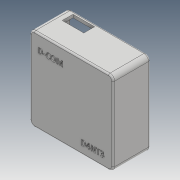
# Autodesk Inventor part: base
Saved by Autodesk Inventor 2017 (Build 210142000, 142)
## iProperties
Created: 2020-06-11
Part Number: base
Material: Generic
Document SubType Name: Modeling
Designer: c
Density: 1 g/cm^3
Appearance: Default
Author: c
Autodesk Inventor part; units mm, degrees
ref_plane "YZ Plane" through (0, 0, 0) normal (1, 0, 0) x (0, 1, 0)
ref_plane "XZ Plane" through (0, 0, 0) normal (0, 1, 0) x (-1, 0, 0)
ref_plane "XY Plane" through (0, 0, 0) normal (0, 0, 1) x (1, 0, 0)
sketch "Sketch1" plane through (0, 0, 0) normal (0, 1, 0) x (-1, 0, 0)
  line L0 (13, 15) -> (-37, 15)
  line L1 (-37, 15) -> (-37, -35)
  line L2 (-37, -35) -> (13, -35)
  line L3 (13, -35) -> (13, 15)
  line L4 (12, 17) -> (-36, 17)
  line L5 (-39, 14) -> (-39, -34)
  line L6 (-36, -37) -> (12, -37)
  line L7 (15, -34) -> (15, 14)
  arc A0 (15, 14) -> (12, 17) centre (12, 14) ccw
  arc A1 (-36, 17) -> (-39, 14) centre (-36, 14) ccw
  arc A2 (-39, -34) -> (-36, -37) centre (-36, -34) ccw
  arc A3 (12, -37) -> (15, -34) centre (12, -34) ccw
  point P0 (0, 0)
  dimension "d0" = 50
  dimension "d1" = 50
  dimension "d2" = 3
  constraints: 16 end point, 8 point on circle, 8 tangent, 4 centre point, 4 parallel, 3 equal radius, 2 perpendicular, 1 horizontal, 3 other
  measures "d0" distance of L2.end L1.end
  measures "d1" distance of L1.end L0.end
  measures "d2" radius of A0
extrude "Extrusion1" add sketch "Sketch1" along normal blind 24
sketch "Sketch2" plane through (0, 0, 0) normal (0, -1, 0) x (1, 0, 0)
  line L0 (36, 17) -> (-12, 17)
  line L1 (-15, 14) -> (-15, -34)
  line L2 (-12, -37) -> (36, -37)
  line L3 (39, -34) -> (39, 14)
  arc A0 (39, 14) -> (36, 17) centre (36, 14) ccw
  arc A1 (-12, 17) -> (-15, 14) centre (-12, 14) ccw
  arc A2 (-15, -34) -> (-12, -37) centre (-12, -34) ccw
  arc A3 (36, -37) -> (39, -34) centre (36, -34) ccw
  point P0 (0, 0)
  dimension "d5" = 3
  constraints: 8 end point, 8 point on circle, 8 tangent, 4 centre point, 3 equal radius, 2 parallel, 1 horizontal, 1 perpendicular
  measures "d5" radius of A0
extrude "Extrusion2" add sketch "Sketch2" against normal blind 2
fillet "Fillet1" radius 1 8 edges at (-14.1213, 0, 16.1213) (-15, 0, -10) (-14.1213, 0, -36.1213) (12, 0, -37) (38.1213, 0, -36.1213) (39, 0, -10) (38.1213, 0, 16.1213) (12, 0, 17)
sketch "Sketch3" plane through (36, 24, -37) normal (0, 0, -1) x (-1, 0, 0)
  line L0 (29, -12) -> (19, -12)
  line L1 (19, -12) -> (19, -8)
  line L2 (19, -8) -> (29, -8)
  line L3 (29, -8) -> (29, -12)
  line L4 (29, -18) -> (19, -18)
  line L5 (19, -18) -> (19, -14)
  line L6 (19, -14) -> (29, -14)
  line L7 (29, -14) -> (29, -18)
  line L8 (0, 0) -> (48, 0) projected
  line L9 (51, -23) -> (51, 0) projected
  line L10 (0, -24) -> (48, -24) projected
  point P0 (36, -24)
  dimension "d9" = 10
  dimension "d10" = 4
  dimension "d11" = 10
  dimension "d12" = 2
  dimension "d16" = 22
  dimension "d17" = 4
  dimension "d25" = 10
  constraints: 16 end point, 4 parallel, 2 horizontal, 2 perpendicular, 1 point on line
  measures "d9" distance of L1.end L2.end
  measures "d10" distance of L0.end L1.end
  measures "d11" distance of L5.end L6.end
  measures "d12" distance between parallel lines of L0 L6
  measures "d16" distance between parallel lines of L9 L7
  measures "d17" distance of L4.end L5.end
  measures "d25" distance between parallel lines of L10 L6
extrude "Extrusion3" cut sketch "Sketch3" against normal blind 4
sketch "Sketch4" plane through (0, 0, 0) normal (0, -1, 0) x (1, 0, 0)
  line L0 (18.0093, -28.2459) -> (38.9151, -28.2459) construction
  line L1 (38.9151, -28.2459) -> (38.9151, -38.6095) construction
  line L2 (38.9151, -38.6095) -> (18.0093, -38.6095) construction
  line L3 (18.0093, -38.6095) -> (18.0093, -28.2459) construction
  line L4 (-9.7906, 9.4463) -> (11.1152, 9.4463) construction
  line L5 (11.1152, 9.4463) -> (11.1152, -33.5941) construction
  line L6 (11.1152, -33.5941) -> (-9.7906, -33.5941) construction
  line L7 (-9.7906, -33.5941) -> (-9.7906, 9.4463) construction
  spline S0 degree 2 poles (21.2858, -29.9976) (21.2858, -30.4774) (21.0361, -31.1577) (20.5661, -31.5915) (19.8957, -31.7919) (19.4323, -31.7919) knots 0 0 0 1 2 3 4 4 4
  line L8 (19.4323, -31.7919) -> (18.6009, -31.7919)
  spline S1 degree 2 poles (18.6009, -31.7919) (18.5121, -31.7919) (18.3905, -31.6868) (18.3905, -31.5685) knots 0 0 0 1 2 2 2
  line L9 (18.3905, -31.5685) -> (18.3905, -28.5319)
  spline S2 degree 2 poles (18.3905, -28.5319) (18.3905, -28.4135) (18.5121, -28.3084) (18.6009, -28.3084) knots 0 0 0 1 2 2 2
  line L10 (18.6009, -28.3084) -> (19.4948, -28.3084)
  spline S3 degree 2 poles (19.4948, -28.3084) (19.9614, -28.3084) (20.6088, -28.5253) (21.0558, -28.9558) (21.2858, -29.5835) (21.2858, -29.9976) knots 0 0 0 1 2 3 4 4 4
  spline S4 degree 2 poles (20.553, -30.0239) (20.553, -29.7774) (20.4379, -29.3502) (20.1816, -29.038) (19.7807, -28.8638) (19.4553, -28.8638) knots 0 0 0 1 2 3 4 4 4
  line L11 (19.4553, -28.8638) -> (19.0971, -28.8638)
  line L12 (19.0971, -28.8638) -> (19.0971, -31.2333)
  line L13 (19.0971, -31.2333) -> (19.4652, -31.2333)
  spline S5 degree 2 poles (19.4652, -31.2333) (19.7577, -31.2333) (20.1553, -31.0821) (20.4215, -30.7797) (20.553, -30.3262) (20.553, -30.0239) knots 0 0 0 1 2 3 4 4 4
  spline S6 degree 2 poles (24.1713, -30.7929) (24.1713, -30.9309) (24.1154, -31.0722) (24.0661, -31.0722) knots 0 0 0 1 2 2 2
  line L14 (24.0661, -31.0722) -> (23.7572, -31.0722)
  line L15 (23.7572, -31.0722) -> (23.7572, -31.6999)
  spline S7 degree 2 poles (23.7572, -31.6999) (23.7572, -31.7262) (23.7243, -31.7689) (23.6455, -31.7952) (23.514, -31.8084) (23.4121, -31.8084) knots 0 0 0 1 2 3 4 4 4
  spline S8 degree 2 poles (23.4121, -31.8084) (23.3168, -31.8084) (23.1854, -31.7952) (23.1065, -31.7689) (23.0769, -31.7262) (23.0769, -31.6999) knots 0 0 0 1 2 3 4 4 4
  line L16 (23.0769, -31.6999) -> (23.0769, -31.0722)
  line L17 (23.0769, -31.0722) -> (21.7426, -31.0722)
  spline S9 degree 2 poles (21.7426, -31.0722) (21.7032, -31.0722) (21.6441, -31.0525) (21.6046, -30.9868) (21.5849, -30.8586) (21.5849, -30.7535) knots 0 0 0 1 2 3 4 4 4
  spline S10 degree 2 poles (21.5849, -30.7535) (21.5849, -30.668) (21.5915, -30.5431) (21.6112, -30.438) (21.6473, -30.3492) (21.6736, -30.2966) knots 0 0 0 1 2 3 4 4 4
  line L18 (21.6736, -30.2966) -> (22.7581, -28.3873)
  spline S11 degree 2 poles (22.7581, -28.3873) (22.7713, -28.361) (22.837, -28.3281) (22.952, -28.3018) (23.1295, -28.2919) (23.2577, -28.2919) knots 0 0 0 1 2 3 4 4 4
  spline S12 degree 2 poles (23.2577, -28.2919) (23.3957, -28.2919) (23.5863, -28.3051) (23.7046, -28.3347) (23.7572, -28.3774) (23.7572, -28.407) knots 0 0 0 1 2 3 4 4 4
  line L19 (23.7572, -28.407) -> (23.7572, -30.507)
  line L20 (23.7572, -30.507) -> (24.0661, -30.507)
  spline S13 degree 2 poles (24.0661, -30.507) (24.1088, -30.507) (24.1713, -30.6384) (24.1713, -30.7929) knots 0 0 0 1 2 2 2
  line L21 (23.0769, -28.9032) -> (23.0703, -28.9032)
  line L22 (23.0703, -28.9032) -> (22.1502, -30.507)
  line L23 (22.1502, -30.507) -> (23.0769, -30.507)
  line L24 (23.0769, -30.507) -> (23.0769, -28.9032)
  spline S14 degree 2 poles (27.5333, -31.5455) (27.5333, -31.6079) (27.4905, -31.7032) (27.4182, -31.7689) (27.3164, -31.7985) (27.2671, -31.7985) knots 0 0 0 1 2 3 4 4 4
  line L25 (27.2671, -31.7985) -> (26.9647, -31.7985)
  spline S15 degree 2 poles (26.9647, -31.7985) (26.8727, -31.7985) (26.7347, -31.7591) (26.6196, -31.6605) (26.5112, -31.4896) (26.4422, -31.3581) knots 0 0 0 1 2 3 4 4 4
  line L26 (26.4422, -31.3581) -> (25.5746, -29.7281)
  spline S16 degree 2 poles (25.5746, -29.7281) (25.499, -29.5835) (25.3445, -29.245) (25.2821, -29.0873) knots 0 0 0 1 2 2 2
  line L27 (25.2821, -29.0873) -> (25.2755, -29.0873)
  spline S17 degree 2 poles (25.2755, -29.0873) (25.2887, -29.2812) (25.2985, -29.6657) (25.2985, -29.8694) knots 0 0 0 1 2 2 2
  line L28 (25.2985, -29.8694) -> (25.2985, -31.6934)
  spline S18 degree 2 poles (25.2985, -31.6934) (25.2985, -31.7196) (25.2689, -31.7624) (25.1966, -31.7919) (25.0718, -31.8084) (24.9764, -31.8084) knots 0 0 0 1 2 3 4 4 4
  spline S19 degree 2 poles (24.9764, -31.8084) (24.8811, -31.8084) (24.7563, -31.7919) (24.6872, -31.7624) (24.661, -31.7196) (24.661, -31.6934) knots 0 0 0 1 2 3 4 4 4
  line L29 (24.661, -31.6934) -> (24.661, -28.5614)
  spline S20 degree 2 poles (24.661, -28.5614) (24.661, -28.4333) (24.8088, -28.3084) (24.9173, -28.3084) knots 0 0 0 1 2 2 2
  line L30 (24.9173, -28.3084) -> (25.2952, -28.3084)
  spline S21 degree 2 poles (25.2952, -28.3084) (25.3971, -28.3084) (25.5384, -28.3445) (25.6469, -28.4234) (25.7455, -28.568) (25.798, -28.6732) knots 0 0 0 1 2 3 4 4 4
  line L31 (25.798, -28.6732) -> (26.475, -29.945)
  spline S22 degree 2 poles (26.475, -29.945) (26.5342, -30.0633) (26.6492, -30.2868) (26.7577, -30.5103) (26.8595, -30.7239) (26.9088, -30.8323) knots 0 0 0 1 2 3 4 4 4
  line L32 (26.9088, -30.8323) -> (26.9121, -30.8323)
  spline S23 degree 2 poles (26.9121, -30.8323) (26.9023, -30.645) (26.8957, -30.2342) (26.8957, -30.0469) knots 0 0 0 1 2 2 2
  line L33 (26.8957, -30.0469) -> (26.8957, -28.4103)
  spline S24 degree 2 poles (26.8957, -28.4103) (26.8957, -28.384) (26.9286, -28.3412) (27.0041, -28.3084) (27.1257, -28.2952) (27.2243, -28.2952) knots 0 0 0 1 2 3 4 4 4
  spline S25 degree 2 poles (27.2243, -28.2952) (27.3164, -28.2952) (27.4379, -28.3084) (27.507, -28.3412) (27.5333, -28.384) (27.5333, -28.4103) knots 0 0 0 1 2 3 4 4 4
  line L34 (27.5333, -28.4103) -> (27.5333, -31.5455)
  spline S26 degree 2 poles (30.606, -28.5976) (30.606, -28.6765) (30.5929, -28.7882) (30.5666, -28.8539) (30.5239, -28.8868) (30.5009, -28.8868) knots 0 0 0 1 2 3 4 4 4
  line L35 (30.5009, -28.8868) -> (29.63, -28.8868)
  line L36 (29.63, -28.8868) -> (29.63, -31.6966)
  spline S27 degree 2 poles (29.63, -31.6966) (29.63, -31.7229) (29.5938, -31.7657) (29.5149, -31.7919) (29.3769, -31.8084) (29.275, -31.8084) knots 0 0 0 1 2 3 4 4 4
  spline S28 degree 2 poles (29.275, -31.8084) (29.1732, -31.8084) (29.0351, -31.7919) (28.9563, -31.7657) (28.9201, -31.7229) (28.9201, -31.6966) knots 0 0 0 1 2 3 4 4 4
  line L37 (28.9201, -31.6966) -> (28.9201, -28.8868)
  line L38 (28.9201, -28.8868) -> (28.0492, -28.8868)
  spline S29 degree 2 poles (28.0492, -28.8868) (28.0229, -28.8868) (27.9835, -28.8539) (27.9572, -28.7882) (27.9441, -28.6765) (27.9441, -28.5976) knots 0 0 0 1 2 3 4 4 4
  spline S30 degree 2 poles (27.9441, -28.5976) (27.9441, -28.5187) (27.9572, -28.4037) (27.9835, -28.338) (28.0229, -28.3084) (28.0492, -28.3084) knots 0 0 0 1 2 3 4 4 4
  line L39 (28.0492, -28.3084) -> (30.5009, -28.3084)
  spline S31 degree 2 poles (30.5009, -28.3084) (30.5239, -28.3084) (30.5666, -28.338) (30.5929, -28.4037) (30.606, -28.5187) (30.606, -28.5976) knots 0 0 0 1 2 3 4 4 4
  spline S32 degree 2 poles (33.2023, -30.7732) (33.2023, -31.0328) (33.0018, -31.437) (32.6469, -31.7131) (32.1506, -31.8544) (31.8581, -31.8544) knots 0 0 0 1 2 3 4 4 4
  spline S33 degree 2 poles (31.8581, -31.8544) (31.6807, -31.8544) (31.3685, -31.8018) (31.1286, -31.7295) (30.9708, -31.6473) (30.9248, -31.6046) (30.8985, -31.5488) (30.8788, -31.4765) (30.8722, -31.368) (30.8722, -31.2891) knots 0 0 0 1 2 3 4 5 6 7 8 8 8
  spline S34 degree 2 poles (30.8722, -31.2891) (30.8722, -31.1577) (30.9149, -31.0591) (30.9577, -31.0591) knots 0 0 0 1 2 2 2
  spline S35 degree 2 poles (30.9577, -31.0591) (30.984, -31.0591) (31.1187, -31.1314) (31.3225, -31.2168) (31.5985, -31.2891) (31.7727, -31.2891) knots 0 0 0 1 2 3 4 4 4
  spline S36 degree 2 poles (31.7727, -31.2891) (31.9206, -31.2891) (32.1473, -31.2201) (32.3051, -31.0919) (32.384, -30.9112) (32.384, -30.8027) knots 0 0 0 1 2 3 4 4 4
  spline S37 degree 2 poles (32.384, -30.8027) (32.384, -30.6812) (32.2887, -30.4873) (32.1046, -30.3492) (31.822, -30.2736) (31.6281, -30.2736) knots 0 0 0 1 2 3 4 4 4
  line L40 (31.6281, -30.2736) -> (31.3257, -30.2736)
  spline S38 degree 2 poles (31.3257, -30.2736) (31.2929, -30.2736) (31.2436, -30.2539) (31.2107, -30.1948) (31.1976, -30.0896) (31.1976, -30.0074) knots 0 0 0 1 2 3 4 4 4
  spline S39 degree 2 poles (31.1976, -30.0074) (31.1976, -29.9286) (31.2107, -29.83) (31.2403, -29.7774) (31.2863, -29.7544) (31.3192, -29.7544) knots 0 0 0 1 2 3 4 4 4
  line L41 (31.3192, -29.7544) -> (31.6248, -29.7544)
  spline S40 degree 2 poles (31.6248, -29.7544) (31.7825, -29.7544) (32.0257, -29.6821) (32.1901, -29.5473) (32.2755, -29.3567) (32.2755, -29.2384) knots 0 0 0 1 2 3 4 4 4
  spline S41 degree 2 poles (32.2755, -29.2384) (32.2755, -29.1497) (32.2164, -28.9919) (32.1013, -28.8769) (31.9173, -28.8079) (31.7924, -28.8079) knots 0 0 0 1 2 3 4 4 4
  spline S42 degree 2 poles (31.7924, -28.8079) (31.6511, -28.8079) (31.4046, -28.8901) (31.2074, -28.9919) (31.0694, -29.0774) (31.0365, -29.0774) knots 0 0 0 1 2 3 4 4 4
  spline S43 degree 2 poles (31.0365, -29.0774) (31.0168, -29.0774) (30.984, -29.0577) (30.961, -29.0051) (30.9511, -28.9032) (30.9511, -28.8211) knots 0 0 0 1 2 3 4 4 4
  spline S44 degree 2 poles (30.9511, -28.8211) (30.9511, -28.7553) (30.9577, -28.6666) (30.9741, -28.6074) (30.9971, -28.5647) (31.0497, -28.5121) (31.2173, -28.4103) (31.4703, -28.3117) (31.8023, -28.2459) (31.9962, -28.2459) knots 0 0 0 1 2 3 4 5 6 7 8 8 8
  spline S45 degree 2 poles (31.9962, -28.2459) (32.2492, -28.2459) (32.6403, -28.3642) (32.9065, -28.5877) (33.0445, -28.9131) (33.0445, -29.1201) knots 0 0 0 1 2 3 4 4 4
  spline S46 degree 2 poles (33.0445, -29.1201) (33.0445, -29.2779) (32.9624, -29.5506) (32.8079, -29.7675) (32.5713, -29.9187) (32.4201, -29.9549) knots 0 0 0 1 2 3 4 4 4
  line L42 (32.4201, -29.9549) -> (32.4201, -29.9647)
  spline S47 degree 2 poles (32.4201, -29.9647) (32.6009, -29.9844) (32.8933, -30.129) (33.0938, -30.3427) (33.2023, -30.6154) (33.2023, -30.7732) knots 0 0 0 1 2 3 4 4 4
  spline S48 degree 2 poles (-6.5141, 7.6946) (-6.5141, 7.2148) (-6.7638, 6.5345) (-7.2338, 6.1007) (-7.9042, 5.9002) (-8.3676, 5.9002) knots 0 0 0 1 2 3 4 4 4
  line L43 (-8.3676, 5.9002) -> (-9.1991, 5.9002)
  spline S49 degree 2 poles (-9.1991, 5.9002) (-9.2878, 5.9002) (-9.4094, 6.0054) (-9.4094, 6.1237) knots 0 0 0 1 2 2 2
  line L44 (-9.4094, 6.1237) -> (-9.4094, 9.1603)
  spline S50 degree 2 poles (-9.4094, 9.1603) (-9.4094, 9.2786) (-9.2878, 9.3838) (-9.1991, 9.3838) knots 0 0 0 1 2 2 2
  line L45 (-9.1991, 9.3838) -> (-8.3052, 9.3838)
  spline S51 degree 2 poles (-8.3052, 9.3838) (-7.8385, 9.3838) (-7.1911, 9.1669) (-6.7441, 8.7364) (-6.5141, 8.1087) (-6.5141, 7.6946) knots 0 0 0 1 2 3 4 4 4
  spline S52 degree 2 poles (-7.2469, 7.6683) (-7.2469, 7.9148) (-7.362, 8.342) (-7.6183, 8.6542) (-8.0192, 8.8284) (-8.3446, 8.8284) knots 0 0 0 1 2 3 4 4 4
  line L46 (-8.3446, 8.8284) -> (-8.7028, 8.8284)
  line L47 (-8.7028, 8.8284) -> (-8.7028, 6.4589)
  line L48 (-8.7028, 6.4589) -> (-8.3347, 6.4589)
  spline S53 degree 2 poles (-8.3347, 6.4589) (-8.0422, 6.4589) (-7.6446, 6.6101) (-7.3784, 6.9125) (-7.2469, 7.366) (-7.2469, 7.6683) knots 0 0 0 1 2 3 4 4 4
  spline S54 degree 2 poles (-4.7854, 7.2542) (-4.7854, 7.0998) (-4.8446, 6.9749) (-4.9103, 6.9749) knots 0 0 0 1 2 2 2
  line L49 (-4.9103, 6.9749) -> (-6.0277, 6.9749)
  spline S55 degree 2 poles (-6.0277, 6.9749) (-6.0967, 6.9749) (-6.1559, 7.1031) (-6.1559, 7.2542) knots 0 0 0 1 2 2 2
  spline S56 degree 2 poles (-6.1559, 7.2542) (-6.1559, 7.4054) (-6.0967, 7.5303) (-6.0277, 7.5303) knots 0 0 0 1 2 2 2
  line L50 (-6.0277, 7.5303) -> (-4.9103, 7.5303)
  spline S57 degree 2 poles (-4.9103, 7.5303) (-4.8775, 7.5303) (-4.8314, 7.504) (-4.7986, 7.4383) (-4.7854, 7.3298) (-4.7854, 7.2542) knots 0 0 0 1 2 3 4 4 4
  spline S58 degree 2 poles (-1.8343, 6.4294) (-1.8343, 6.3636) (-1.8408, 6.2683) (-1.8573, 6.2026) (-1.8868, 6.1533) (-1.946, 6.0909) (-2.1136, 5.9923) (-2.3601, 5.9035) (-2.6756, 5.8444) (-2.8563, 5.8444) knots 0 0 0 1 2 3 4 5 6 7 8 8 8
  spline S59 degree 2 poles (-2.8563, 5.8444) (-3.2145, 5.8444) (-3.7929, 6.0646) (-4.1939, 6.5049) (-4.4108, 7.1589) (-4.4108, 7.596) knots 0 0 0 1 2 3 4 4 4
  spline S60 degree 2 poles (-4.4108, 7.596) (-4.4108, 8.0397) (-4.1742, 8.7298) (-3.7469, 9.1965) (-3.1521, 9.4397) (-2.7939, 9.4397) knots 0 0 0 1 2 3 4 4 4
  spline S61 degree 2 poles (-2.7939, 9.4397) (-2.6493, 9.4397) (-2.3798, 9.3904) (-2.1498, 9.3115) (-1.969, 9.2096) (-1.8967, 9.1373) (-1.8671, 9.088) (-1.8507, 9.0125) (-1.8441, 8.9106) (-1.8441, 8.835) knots 0 0 0 1 2 3 4 5 6 7 8 8 8
  spline S62 degree 2 poles (-1.8441, 8.835) (-1.8441, 8.7561) (-1.854, 8.6411) (-1.8803, 8.5721) (-1.9197, 8.5392) (-1.9427, 8.5392) knots 0 0 0 1 2 3 4 4 4
  spline S63 degree 2 poles (-1.9427, 8.5392) (-1.9854, 8.5392) (-2.107, 8.6345) (-2.3042, 8.7495) (-2.577, 8.8448) (-2.7643, 8.8448) knots 0 0 0 1 2 3 4 4 4
  spline S64 degree 2 poles (-2.7643, 8.8448) (-2.9714, 8.8448) (-3.2967, 8.674) (-3.5268, 8.3617) (-3.6451, 7.9148) (-3.6451, 7.6355) knots 0 0 0 1 2 3 4 4 4
  spline S65 degree 2 poles (-3.6451, 7.6355) (-3.6451, 7.3265) (-3.5202, 6.8796) (-3.2836, 6.5871) (-2.9549, 6.4458) (-2.7479, 6.4458) knots 0 0 0 1 2 3 4 4 4
  spline S66 degree 2 poles (-2.7479, 6.4458) (-2.5573, 6.4458) (-2.2845, 6.5345) (-2.0873, 6.643) (-1.9591, 6.7284) (-1.9263, 6.7284) knots 0 0 0 1 2 3 4 4 4
  spline S67 degree 2 poles (-1.9263, 6.7284) (-1.9, 6.7284) (-1.8671, 6.7054) (-1.8441, 6.643) (-1.8343, 6.5279) (-1.8343, 6.4294) knots 0 0 0 1 2 3 4 4 4
  spline S68 degree 2 poles (1.8103, 7.6815) (1.8103, 7.2477) (1.5934, 6.5641) (1.1695, 6.0876) (0.5418, 5.8378) (0.131, 5.8378) knots 0 0 0 1 2 3 4 4 4
  spline S69 degree 2 poles (0.131, 5.8378) (-0.2765, 5.8378) (-0.8845, 6.0514) (-1.2887, 6.4852) (-1.4892, 7.1589) (-1.4892, 7.619) knots 0 0 0 1 2 3 4 4 4
  spline S70 degree 2 poles (-1.4892, 7.619) (-1.4892, 8.043) (-1.2723, 8.72) (-0.8483, 9.1932) (-0.2206, 9.4463) (0.1934, 9.4463) knots 0 0 0 1 2 3 4 4 4
  spline S71 degree 2 poles (0.1934, 9.4463) (0.5911, 9.4463) (1.1958, 9.2359) (1.6033, 8.7988) (1.8103, 8.135) (1.8103, 7.6815) knots 0 0 0 1 2 3 4 4 4
  spline S72 degree 2 poles (1.0676, 7.6453) (1.0676, 7.9181) (0.9822, 8.3683) (0.7751, 8.6904) (0.4301, 8.8646) (0.1704, 8.8646) knots 0 0 0 1 2 3 4 4 4
  spline S73 degree 2 poles (0.1704, 8.8646) (-0.0925, 8.8646) (-0.4408, 8.6674) (-0.6577, 8.3387) (-0.7465, 7.9017) (-0.7465, 7.6552) knots 0 0 0 1 2 3 4 4 4
  spline S74 degree 2 poles (-0.7465, 7.6552) (-0.7465, 7.3693) (-0.661, 6.9157) (-0.454, 6.5937) (-0.1089, 6.4228) (0.1507, 6.4228) knots 0 0 0 1 2 3 4 4 4
  spline S75 degree 2 poles (0.1507, 6.4228) (0.4136, 6.4228) (0.762, 6.6167) (0.9789, 6.9519) (1.0676, 7.3955) (1.0676, 7.6453) knots 0 0 0 1 2 3 4 4 4
  spline S76 degree 2 poles (6.4671, 5.9955) (6.4671, 5.9693) (6.4376, 5.9265) (6.3587, 5.9002) (6.2305, 5.8838) (6.1319, 5.8838) knots 0 0 0 1 2 3 4 4 4
  spline S77 degree 2 poles (6.1319, 5.8838) (6.0333, 5.8838) (5.9052, 5.9002) (5.8296, 5.9265) (5.7967, 5.9693) (5.7967, 5.9955) knots 0 0 0 1 2 3 4 4 4
  line L51 (5.7967, 5.9955) -> (5.7967, 8.8317)
  line L52 (5.7967, 8.8317) -> (5.7902, 8.8317)
  line L53 (5.7902, 8.8317) -> (4.7812, 5.9988)
  spline S78 degree 2 poles (4.7812, 5.9988) (4.7714, 5.966) (4.7221, 5.92) (4.6399, 5.8904) (4.5085, 5.8838) (4.4164, 5.8838) knots 0 0 0 1 2 3 4 4 4
  spline S79 degree 2 poles (4.4164, 5.8838) (4.3277, 5.8838) (4.1963, 5.897) (4.1141, 5.9265) (4.0648, 5.9693) (4.0582, 5.9988) knots 0 0 0 1 2 3 4 4 4
  line L54 (4.0582, 5.9988) -> (3.0822, 8.8317)
  line L55 (3.0822, 8.8317) -> (3.0756, 8.8317)
  line L56 (3.0756, 8.8317) -> (3.0756, 5.9955)
  spline S80 degree 2 poles (3.0756, 5.9955) (3.0756, 5.9693) (3.046, 5.9265) (2.9639, 5.9002) (2.839, 5.8838) (2.7404, 5.8838) knots 0 0 0 1 2 3 4 4 4
  spline S81 degree 2 poles (2.7404, 5.8838) (2.6418, 5.8838) (2.5136, 5.9002) (2.4348, 5.9265) (2.4052, 5.9693) (2.4052, 5.9955) knots 0 0 0 1 2 3 4 4 4
  line L57 (2.4052, 5.9955) -> (2.4052, 9.1012)
  spline S82 degree 2 poles (2.4052, 9.1012) (2.4052, 9.2392) (2.5498, 9.3838) (2.6714, 9.3838) knots 0 0 0 1 2 2 2
  line L58 (2.6714, 9.3838) -> (3.1348, 9.3838)
  spline S83 degree 2 poles (3.1348, 9.3838) (3.2596, 9.3838) (3.4371, 9.3444) (3.5653, 9.2491) (3.6507, 9.0946) (3.6836, 8.9829) knots 0 0 0 1 2 3 4 4 4
  line L59 (3.6836, 8.9829) -> (4.4394, 6.9059)
  line L60 (4.4394, 6.9059) -> (4.4493, 6.9059)
  line L61 (4.4493, 6.9059) -> (5.2315, 8.9763)
  spline S84 degree 2 poles (5.2315, 8.9763) (5.2676, 9.0913) (5.3498, 9.2458) (5.4615, 9.3444) (5.6094, 9.3838) (5.7113, 9.3838) knots 0 0 0 1 2 3 4 4 4
  line L62 (5.7113, 9.3838) -> (6.1878, 9.3838)
  spline S85 degree 2 poles (6.1878, 9.3838) (6.2601, 9.3838) (6.3653, 9.3477) (6.431, 9.2721) (6.4671, 9.1669) (6.4671, 9.1012) knots 0 0 0 1 2 3 4 4 4
  line L63 (6.4671, 9.1012) -> (6.4671, 5.9955)
  point P0 (0, 0)
  constraints: 4 other
emboss "Emboss1" sketch "Sketch4" operation cut depth 1 direction (0, 1, 0)
sketch "Sketch5" plane through (-12, 24, 17) normal (0, 0, 1) x (1, 0, 0)
  line L0 (29, -12) -> (29, -8) projected
  line L1 (17, -9) -> (2.9977, -9)
  line L2 (2.9977, -9) -> (2.9977, -2)
  line L3 (2.9977, -2) -> (17, -2)
  line L4 (17, -2) -> (17, -9)
  line L5 (-3, -23) -> (-3, 0) projected
  line L6 (0, -24) -> (48, -24) projected
  point P0 (12, -24)
  dimension "d26" = 20
  dimension "d27" = 15
  dimension "d28" = 7
  constraints: 8 end point, 2 parallel, 1 horizontal, 1 perpendicular
  measures "d26" distance between parallel lines of L5 L4
  measures "d27" distance between parallel lines of L6 L1
  measures "d28" distance between parallel lines of L1 L3
extrude "Extrusion4" cut sketch "Sketch5" against normal blind 4
fillet "Fillet2" radius 1 8 edges at (38.1213, 24, 16.1213) (39, 24, -10) (38.1213, 24, -36.1213) (12, 24, -37) (-14.1213, 24, -36.1213) (-15, 24, -10) (-14.1213, 24, 16.1213) (12, 24, 17)
sketch "Sketch6" plane through (36, 1, -37) normal (0, 0, -1) x (-1, 0, 0)
  line L0 (12.8463, 14.3019) -> (16.3491, 14.3019) construction
  line L1 (16.3491, 14.3019) -> (16.3491, 11.5535) construction
  line L2 (16.3491, 11.5535) -> (12.8463, 11.5535) construction
  line L3 (12.8463, 11.5535) -> (12.8463, 14.3019) construction
  line L4 (14.0879, 6.9979) -> (15.9812, 6.9979) construction
  line L5 (15.9812, 6.9979) -> (15.9812, 0.7326) construction
  line L6 (15.9812, 0.7326) -> (14.0879, 0.7326) construction
  line L7 (14.0879, 0.7326) -> (14.0879, 6.9979) construction
  line L8 (15.9804, 12.7391) -> (14.7948, 12.7391)
  line L9 (14.7948, 12.7391) -> (14.7948, 11.5535)
  line L10 (14.7948, 11.5535) -> (14.4034, 11.5535)
  line L11 (14.4034, 11.5535) -> (14.4034, 12.7391)
  line L12 (14.4034, 12.7391) -> (13.2178, 12.7391)
  line L13 (13.2178, 12.7391) -> (13.2178, 13.1163)
  line L14 (13.2178, 13.1163) -> (14.4034, 13.1163)
  line L15 (14.4034, 13.1163) -> (14.4034, 14.3019)
  line L16 (14.4034, 14.3019) -> (14.7948, 14.3019)
  line L17 (14.7948, 14.3019) -> (14.7948, 13.1163)
  line L18 (14.7948, 13.1163) -> (15.9804, 13.1163)
  line L19 (15.9804, 13.1163) -> (15.9804, 12.7391)
  line L20 (15.6252, 6.5725) -> (14.3007, 6.5725)
  line L21 (14.3007, 6.5725) -> (14.3007, 6.9979)
  line L22 (14.3007, 6.9979) -> (15.6252, 6.9979)
  line L23 (15.6252, 6.9979) -> (15.6252, 6.5725)
  point P0 (36, -1)
  constraints: 4 other
emboss "Emboss2" sketch "Sketch6" operation cut depth 1 direction (0, 0, 1)
body "Solid1"
